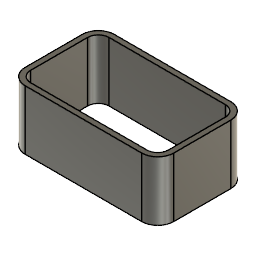
▢-200×150×9.0 (Autodesk Fusion 360 design; units mm, degrees)
Autodesk Fusion 360 part; units mm, degrees
sketch "スケッチ1" plane through (0, 0, 0) normal (0, 0, 1) x (1, 0, 0)
  line L0 (1019.5693, -278.9332) -> (1215.5693, -278.9332)
  line L1 (1019.5693, -269.9332) -> (1215.5693, -269.9332)
  line L2 (1215.5693, -128.9332) -> (1019.5693, -128.9332)
  line L3 (1215.5693, -137.9332) -> (1019.5693, -137.9332)
  arc A0 (992.5693, -251.9332) -> (1019.5693, -278.9332) centre (1019.5693, -251.9332) ccw
  arc A1 (1001.5693, -251.9332) -> (1019.5693, -269.9332) centre (1019.5693, -251.9332) ccw
  line L4 (992.5693, -155.9332) -> (992.5693, -251.9332)
  line L5 (1001.5693, -155.9332) -> (1001.5693, -251.9332)
  arc A2 (1019.5693, -128.9332) -> (992.5693, -155.9332) centre (1019.5693, -155.9332) ccw
  arc A3 (1019.5693, -137.9332) -> (1001.5693, -155.9332) centre (1019.5693, -155.9332) ccw
  arc A4 (1215.5693, -278.9332) -> (1242.5693, -251.9332) centre (1215.5693, -251.9332) ccw
  arc A5 (1215.5693, -269.9332) -> (1233.5693, -251.9332) centre (1215.5693, -251.9332) ccw
  line L6 (1242.5693, -251.9332) -> (1242.5693, -155.9332)
  line L7 (1233.5693, -251.9332) -> (1233.5693, -155.9332)
  arc A6 (1242.5693, -155.9332) -> (1215.5693, -128.9332) centre (1215.5693, -155.9332) ccw
  arc A7 (1233.5693, -155.9332) -> (1215.5693, -137.9332) centre (1215.5693, -155.9332) ccw
  point P0 (1117.5693, -203.9332)
extrude "押し出し1" add sketch "スケッチ1" along normal blind 100
